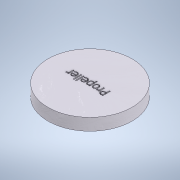
# Autodesk Inventor part: FORS phone case- propeller
Saved by Autodesk Inventor 2021 (Build 250183000, 183)
## iProperties
Created: 2020-06-20
Part Number: FORS phone case- propeller
Material: Generic
Document SubType Name: Modeling
Designer: david
Density: 1 g/cm^3
Appearance: Weld - Aluminum
Author: david
Autodesk Inventor part; units mm, degrees
ref_plane "YZ Plane" through (0, 0, 0) normal (1, 0, 0) x (0, 1, 0)
ref_plane "XZ Plane" through (0, 0, 0) normal (0, 1, 0) x (-1, 0, 0)
ref_plane "XY Plane" through (0, 0, 0) normal (0, 0, 1) x (1, 0, 0)
sketch "Sketch1" plane through (0, 0, 0) normal (0, 1, 0) x (-1, 0, 0)
  circle A0 centre (25.6809, -26.8482) radius 17.78
  point P0 (0, 0)
  dimension "d2" = 35.56
  constraints: 1 centre point
  measures "d2" diameter of A0
extrude "Extrusion1" add sketch "Sketch1" along normal blind 5.08
sketch "Sketch2" plane through (-25.6809, 5.08, -26.8482) normal (0, 1, 0) x (1, 0, 0)
  line L0 (7.6794, -2.0675) -> (6.4813, -2.0675) construction
  line L1 (6.4813, -2.0675) -> (6.4813, -2.9851) construction
  line L2 (6.4813, -2.9851) -> (7.6794, -2.9851) construction
  line L3 (7.6794, -2.9851) -> (7.6794, -2.0675) construction
  spline S0 degree 2 poles (5.3509, -0.9688) (5.3509, -0.763) (5.4976, -0.3925) (5.6288, -0.2639) knots 0 0 0 1 2 2 2
  spline S1 degree 2 poles (5.6288, -0.2639) (5.7934, -0.1018) (6.2386, 0.0655) (6.5782, 0.0655) knots 0 0 0 1 2 2 2
  line L4 (6.5782, 0.0655) -> (6.9358, 0.0655)
  line L5 (6.9358, 0.0655) -> (6.9358, 1.249)
  line L6 (6.9358, 1.249) -> (7.3578, 1.249)
  line L7 (7.3578, 1.249) -> (7.3578, -1.926)
  line L8 (7.3578, -1.926) -> (6.5602, -1.926)
  spline S2 degree 2 poles (6.5602, -1.926) (6.2771, -1.926) (5.8809, -1.8333) (5.7291, -1.7278) knots 0 0 0 1 2 2 2
  spline S3 degree 2 poles (5.7291, -1.7278) (5.5516, -1.6069) (5.3509, -1.2338) (5.3509, -0.9688) knots 0 0 0 1 2 2 2
  spline S4 degree 2 poles (5.7909, -0.956) (5.7909, -1.1206) (5.9041, -1.3625) (6.0199, -1.4397) knots 0 0 0 1 2 2 2
  spline S5 degree 2 poles (6.0199, -1.4397) (6.1202, -1.5066) (6.3878, -1.5606) (6.5859, -1.5606) knots 0 0 0 1 2 2 2
  line L9 (6.5859, -1.5606) -> (6.9358, -1.5606)
  line L10 (6.9358, -1.5606) -> (6.9358, -0.2947)
  line L11 (6.9358, -0.2947) -> (6.6477, -0.2947)
  spline S6 degree 2 poles (6.6477, -0.2947) (6.3904, -0.2947) (6.0739, -0.3771) (5.971, -0.4851) knots 0 0 0 1 2 2 2
  spline S7 degree 2 poles (5.971, -0.4851) (5.8758, -0.5803) (5.7909, -0.8042) (5.7909, -0.956) knots 0 0 0 1 2 2 2
  line L12 (3.7171, -0.7038) -> (3.7377, -0.7038)
  spline S8 degree 2 poles (3.7377, -0.7038) (3.784, -0.7167) (3.8843, -0.7218) (3.9538, -0.7218) knots 0 0 0 1 2 2 2
  spline S9 degree 2 poles (3.9538, -0.7218) (4.1159, -0.7218) (4.4349, -0.5803) (4.579, -0.4414) knots 0 0 0 1 2 2 2
  line L13 (4.579, -0.4414) -> (4.579, 1.249)
  line L14 (4.579, 1.249) -> (4.9804, 1.249)
  line L15 (4.9804, 1.249) -> (4.9804, -1.1335)
  line L16 (4.9804, -1.1335) -> (4.579, -1.1335)
  line L17 (4.579, -1.1335) -> (4.579, -0.7784)
  spline S10 degree 2 poles (4.579, -0.7784) (4.3603, -0.974) (4.0336, -1.1335) (3.8792, -1.1335) knots 0 0 0 1 2 2 2
  spline S11 degree 2 poles (3.8792, -1.1335) (3.8174, -1.1335) (3.7557, -1.1284) (3.7171, -1.1206) knots 0 0 0 1 2 2 2
  line L18 (3.7171, -1.1206) -> (3.7171, -0.7038)
  spline S12 degree 2 poles (1.4478, 0.0578) (1.4478, 0.6598) (2.0267, 1.3159) (2.5104, 1.3159) knots 0 0 0 1 2 2 2
  spline S13 degree 2 poles (2.5104, 1.3159) (3.007, 1.3159) (3.5756, 0.6392) (3.5756, 0.0578) knots 0 0 0 1 2 2 2
  spline S14 degree 2 poles (3.5756, 0.0578) (3.5756, -0.5392) (2.9889, -1.2004) (2.5104, -1.2004) knots 0 0 0 1 2 2 2
  spline S15 degree 2 poles (2.5104, -1.2004) (2.0267, -1.2004) (1.4478, -0.5417) (1.4478, 0.0578) knots 0 0 0 1 2 2 2
  spline S16 degree 2 poles (1.862, 0.0578) (1.862, -0.4054) (2.199, -0.8556) (2.5104, -0.8556) knots 0 0 0 1 2 2 2
  spline S17 degree 2 poles (2.5104, -0.8556) (2.8217, -0.8556) (3.1613, -0.4054) (3.1613, 0.0578) knots 0 0 0 1 2 2 2
  spline S18 degree 2 poles (3.1613, 0.0578) (3.1613, 0.508) (2.8217, 0.9712) (2.5104, 0.9712) knots 0 0 0 1 2 2 2
  spline S19 degree 2 poles (2.5104, 0.9712) (2.2016, 0.9712) (1.862, 0.5157) (1.862, 0.0578) knots 0 0 0 1 2 2 2
  spline S20 degree 2 poles (-0.9605, -0.0066) (-0.9605, 0.5904) (-0.3919, 1.2953) (0.0429, 1.2953) knots 0 0 0 1 2 2 2
  spline S21 degree 2 poles (0.0429, 1.2953) (0.2205, 1.2953) (0.4932, 1.213) (0.6347, 1.1281) knots 0 0 0 1 2 2 2
  line L19 (0.6347, 1.1281) -> (0.6347, 2.1264)
  line L20 (0.6347, 2.1264) -> (1.0361, 2.1264)
  line L21 (1.0361, 2.1264) -> (1.0361, -1.1335)
  line L22 (1.0361, -1.1335) -> (0.6347, -1.1335)
  line L23 (0.6347, -1.1335) -> (0.6347, -0.8839)
  spline S22 degree 2 poles (0.6347, -0.8839) (0.4855, -1.0203) (0.1201, -1.2004) (-0.0934, -1.2004) knots 0 0 0 1 2 2 2
  spline S23 degree 2 poles (-0.0934, -1.2004) (-0.5025, -1.2004) (-0.9605, -0.552) (-0.9605, -0.0066) knots 0 0 0 1 2 2 2
  spline S24 degree 2 poles (-0.5463, 0.0398) (-0.5463, -0.3693) (-0.2864, -0.8196) (0.0043, -0.8196) knots 0 0 0 1 2 2 2
  spline S25 degree 2 poles (0.0043, -0.8196) (0.1742, -0.8196) (0.4932, -0.6678) (0.6347, -0.5494) knots 0 0 0 1 2 2 2
  line L24 (0.6347, -0.5494) -> (0.6347, 0.8039)
  spline S26 degree 2 poles (0.6347, 0.8039) (0.4778, 0.8785) (0.2539, 0.9351) (0.1098, 0.9351) knots 0 0 0 1 2 2 2
  spline S27 degree 2 poles (0.1098, 0.9351) (-0.2015, 0.9351) (-0.5463, 0.4772) (-0.5463, 0.0398) knots 0 0 0 1 2 2 2
  spline S28 degree 2 poles (-2.4116, 1.3031) (-1.8405, 1.3031) (-1.2127, 0.6624) (-1.2127, 0.0706) knots 0 0 0 1 2 2 2
  spline S29 degree 2 poles (-1.2127, 0.0706) (-1.2127, -0.5109) (-1.8224, -1.2004) (-2.3139, -1.2004) knots 0 0 0 1 2 2 2
  spline S30 degree 2 poles (-2.3139, -1.2004) (-2.5351, -1.2004) (-2.8773, -1.0718) (-3.0034, -0.9354) knots 0 0 0 1 2 2 2
  spline S31 degree 2 poles (-3.0034, -0.9354) (-3.1321, -0.799) (-3.2684, -0.4054) (-3.2684, -0.1198) knots 0 0 0 1 2 2 2
  line L25 (-3.2684, -0.1198) -> (-3.2684, 0.0989)
  line L26 (-3.2684, 0.0989) -> (-1.6192, 0.0989)
  spline S32 degree 2 poles (-1.6192, 0.0989) (-1.6192, 0.5132) (-2.036, 0.9531) (-2.4065, 0.9531) knots 0 0 0 1 2 2 2
  spline S33 degree 2 poles (-2.4065, 0.9531) (-2.5377, 0.9531) (-2.7924, 0.894) (-2.8954, 0.8477) knots 0 0 0 1 2 2 2
  spline S34 degree 2 poles (-2.8954, 0.8477) (-3.0034, 0.7962) (-3.1527, 0.7061) (-3.2015, 0.665) knots 0 0 0 1 2 2 2
  line L27 (-3.2015, 0.665) -> (-3.2247, 0.665)
  line L28 (-3.2247, 0.665) -> (-3.2247, 1.1024)
  spline S35 degree 2 poles (-3.2247, 1.1024) (-3.1552, 1.1307) (-2.9442, 1.213) (-2.8619, 1.2362) knots 0 0 0 1 2 2 2
  spline S36 degree 2 poles (-2.8619, 1.2362) (-2.7461, 1.2696) (-2.5557, 1.3031) (-2.4116, 1.3031) knots 0 0 0 1 2 2 2
  spline S37 degree 2 poles (-2.8773, -0.2072) (-2.8722, -0.3693) (-2.8053, -0.6061) (-2.741, -0.6858) knots 0 0 0 1 2 2 2
  spline S38 degree 2 poles (-2.741, -0.6858) (-2.6715, -0.7759) (-2.4528, -0.8711) (-2.2907, -0.8711) knots 0 0 0 1 2 2 2
  spline S39 degree 2 poles (-2.2907, -0.8711) (-2.1312, -0.8711) (-1.9074, -0.7759) (-1.8147, -0.6832) knots 0 0 0 1 2 2 2
  spline S40 degree 2 poles (-1.8147, -0.6832) (-1.7247, -0.588) (-1.632, -0.359) (-1.6192, -0.2072) knots 0 0 0 1 2 2 2
  line L29 (-1.6192, -0.2072) -> (-2.8773, -0.2072)
  line L30 (-4.0841, 1.249) -> (-3.6827, 1.249)
  line L31 (-3.6827, 1.249) -> (-3.6827, -2.0675)
  line L32 (-3.6827, -2.0675) -> (-4.0841, -2.0675)
  line L33 (-4.0841, -2.0675) -> (-4.0841, 1.249)
  line L34 (-5.0824, 1.249) -> (-4.681, 1.249)
  line L35 (-4.681, 1.249) -> (-4.681, -2.0675)
  line L36 (-4.681, -2.0675) -> (-5.0824, -2.0675)
  line L37 (-5.0824, -2.0675) -> (-5.0824, 1.249)
  spline S41 degree 2 poles (-6.7059, 1.3031) (-6.1347, 1.3031) (-5.5069, 0.6624) (-5.5069, 0.0706) knots 0 0 0 1 2 2 2
  spline S42 degree 2 poles (-5.5069, 0.0706) (-5.5069, -0.5109) (-6.1167, -1.2004) (-6.6081, -1.2004) knots 0 0 0 1 2 2 2
  spline S43 degree 2 poles (-6.6081, -1.2004) (-6.8294, -1.2004) (-7.1716, -1.0718) (-7.2976, -0.9354) knots 0 0 0 1 2 2 2
  spline S44 degree 2 poles (-7.2976, -0.9354) (-7.4263, -0.799) (-7.5627, -0.4054) (-7.5627, -0.1198) knots 0 0 0 1 2 2 2
  line L38 (-7.5627, -0.1198) -> (-7.5627, 0.0989)
  line L39 (-7.5627, 0.0989) -> (-5.9134, 0.0989)
  spline S45 degree 2 poles (-5.9134, 0.0989) (-5.9134, 0.5132) (-6.3302, 0.9531) (-6.7007, 0.9531) knots 0 0 0 1 2 2 2
  spline S46 degree 2 poles (-6.7007, 0.9531) (-6.8319, 0.9531) (-7.0867, 0.894) (-7.1896, 0.8477) knots 0 0 0 1 2 2 2
  spline S47 degree 2 poles (-7.1896, 0.8477) (-7.2976, 0.7962) (-7.4469, 0.7061) (-7.4958, 0.665) knots 0 0 0 1 2 2 2
  line L40 (-7.4958, 0.665) -> (-7.5189, 0.665)
  line L41 (-7.5189, 0.665) -> (-7.5189, 1.1024)
  spline S48 degree 2 poles (-7.5189, 1.1024) (-7.4495, 1.1307) (-7.2385, 1.213) (-7.1561, 1.2362) knots 0 0 0 1 2 2 2
  spline S49 degree 2 poles (-7.1561, 1.2362) (-7.0404, 1.2696) (-6.85, 1.3031) (-6.7059, 1.3031) knots 0 0 0 1 2 2 2
  spline S50 degree 2 poles (-7.1716, -0.2072) (-7.1664, -0.3693) (-7.0995, -0.6061) (-7.0352, -0.6858) knots 0 0 0 1 2 2 2
  spline S51 degree 2 poles (-7.0352, -0.6858) (-6.9657, -0.7759) (-6.747, -0.8711) (-6.5849, -0.8711) knots 0 0 0 1 2 2 2
  spline S52 degree 2 poles (-6.5849, -0.8711) (-6.4254, -0.8711) (-6.2016, -0.7759) (-6.109, -0.6832) knots 0 0 0 1 2 2 2
  spline S53 degree 2 poles (-6.109, -0.6832) (-6.0189, -0.588) (-5.9263, -0.359) (-5.9134, -0.2072) knots 0 0 0 1 2 2 2
  line L42 (-5.9134, -0.2072) -> (-7.1716, -0.2072)
  line L43 (-9.2325, -0.7038) -> (-9.2119, -0.7038)
  spline S54 degree 2 poles (-9.2119, -0.7038) (-9.1656, -0.7167) (-9.0653, -0.7218) (-8.9958, -0.7218) knots 0 0 0 1 2 2 2
  spline S55 degree 2 poles (-8.9958, -0.7218) (-8.8337, -0.7218) (-8.5146, -0.5803) (-8.3706, -0.4414) knots 0 0 0 1 2 2 2
  line L44 (-8.3706, -0.4414) -> (-8.3706, 1.249)
  line L45 (-8.3706, 1.249) -> (-7.9692, 1.249)
  line L46 (-7.9692, 1.249) -> (-7.9692, -1.1335)
  line L47 (-7.9692, -1.1335) -> (-8.3706, -1.1335)
  line L48 (-8.3706, -1.1335) -> (-8.3706, -0.7784)
  spline S56 degree 2 poles (-8.3706, -0.7784) (-8.5893, -0.974) (-8.916, -1.1335) (-9.0704, -1.1335) knots 0 0 0 1 2 2 2
  spline S57 degree 2 poles (-9.0704, -1.1335) (-9.1321, -1.1335) (-9.1939, -1.1284) (-9.2325, -1.1206) knots 0 0 0 1 2 2 2
  line L49 (-9.2325, -1.1206) -> (-9.2325, -0.7038)
  point P0 (25.6809, -26.8482)
  constraints: 2 other
emboss "Emboss1" sketch "Sketch2" operation cut depth 2.54 direction (0, -1, 0)
body "Solid1"
